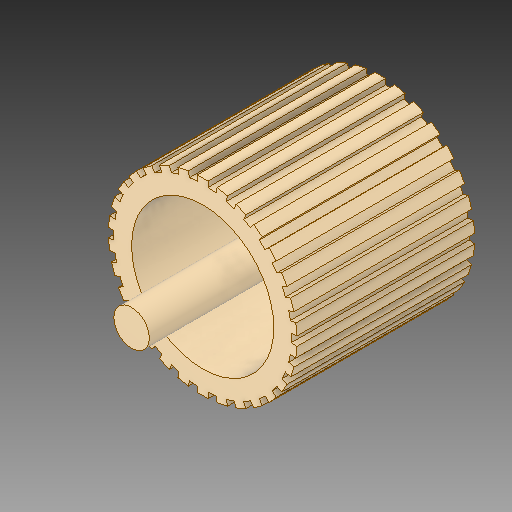
# Autodesk Inventor part: tire
Saved by Autodesk Inventor 2018.1 (Build 221171000, 171)
## iProperties
Created: 2017-10-26
Part Number: tire
Material: 一般
Document SubType Name: Modeling
Designer: Kakeru Yamashita
Density: 28.0819 g/cm^3
Appearance: 滑らか - オフホワイト
Mass: 2000 g
Surface Area: 220.268 cm^2
Volume: 71.2202 cm^3
Author: Kakeru Yamashita
Autodesk Inventor part; units mm, degrees
ref_plane "YZ Plane" through (0, 0, 0) normal (1, 0, 0) x (0, 1, 0)
ref_plane "XZ Plane" through (0, 0, 0) normal (0, 1, 0) x (-1, 0, 0)
ref_plane "XY Plane" through (0, 0, 0) normal (0, 0, 1) x (1, 0, 0)
sketch "スケッチ1" plane through (0, 0, 0) normal (0, 0, 1) x (1, 0, 0)
  line L0 (-37.1163, 0) -> (37.1163, 0) projected
  line L1 (0, -37.1) -> (0, 37.1) projected
  line L2 (1.5, 23.5) -> (1.5, 26.5)
  line L3 (1.5, 26.5) -> (-1.5, 26.5)
  line L4 (-1.5, 26.5) -> (-1.5, 23.5)
  line L5 (-1.5, 23.5) -> (1.5, 23.5)
  line L6 (1.5, 23.5) -> (-1.5, 26.5) construction
  line L7 (1.5, 26.5) -> (-1.5, 23.5) construction
  line L8 (-6.9769, 25.609) -> (-6.3531, 22.6746)
  line L9 (-4.0424, 26.2328) -> (-6.9769, 25.609)
  line L10 (-3.4187, 23.2983) -> (-4.0424, 26.2328)
  line L11 (-6.3531, 22.6746) -> (-3.4187, 23.2983)
  line L12 (-12.1488, 23.5988) -> (-10.9286, 20.8582)
  line L13 (-9.4082, 24.8191) -> (-12.1488, 23.5988)
  line L14 (-8.188, 22.0784) -> (-9.4082, 24.8191)
  line L15 (-10.9286, 20.8582) -> (-8.188, 22.0784)
  line L16 (-16.7898, 20.5573) -> (-15.0265, 18.1302)
  line L17 (-14.3628, 22.3206) -> (-16.7898, 20.5573)
  line L18 (-12.5994, 19.8936) -> (-14.3628, 22.3206)
  line L19 (-15.0265, 18.1302) -> (-12.5994, 19.8936)
  line L20 (-20.697, 16.6172) -> (-18.4676, 14.6099)
  line L21 (-18.6896, 18.8467) -> (-20.697, 16.6172)
  line L22 (-16.4602, 16.8393) -> (-18.6896, 18.8467)
  line L23 (-18.4676, 14.6099) -> (-16.4602, 16.8393)
  line L24 (-23.6997, 11.951) -> (-21.1016, 10.451)
  line L25 (-22.1997, 14.549) -> (-23.6997, 11.951)
  line L26 (-19.6016, 13.049) -> (-22.1997, 14.549)
  line L27 (-21.1016, 10.451) -> (-19.6016, 13.049)
  line L28 (-25.6665, 6.7624) -> (-22.8134, 5.8353)
  line L29 (-24.7395, 9.6155) -> (-25.6665, 6.7624)
  line L30 (-21.8863, 8.6885) -> (-24.7395, 9.6155)
  line L31 (-22.8134, 5.8353) -> (-21.8863, 8.6885)
  line L32 (-26.5116, 1.2782) -> (-23.5281, 0.9646)
  line L33 (-26.198, 4.2618) -> (-26.5116, 1.2782)
  line L34 (-23.2145, 3.9482) -> (-26.198, 4.2618)
  line L35 (-23.5281, 0.9646) -> (-23.2145, 3.9482)
  line L36 (-26.198, -4.2618) -> (-23.2145, -3.9482)
  line L37 (-26.5116, -1.2782) -> (-26.198, -4.2618)
  line L38 (-23.5281, -0.9646) -> (-26.5116, -1.2782)
  line L39 (-23.2145, -3.9482) -> (-23.5281, -0.9646)
  line L40 (-24.7395, -9.6155) -> (-21.8863, -8.6885)
  line L41 (-25.6665, -6.7624) -> (-24.7395, -9.6155)
  line L42 (-22.8134, -5.8353) -> (-25.6665, -6.7624)
  line L43 (-21.8863, -8.6885) -> (-22.8134, -5.8353)
  line L44 (-22.1997, -14.549) -> (-19.6016, -13.049)
  line L45 (-23.6997, -11.951) -> (-22.1997, -14.549)
  line L46 (-21.1016, -10.451) -> (-23.6997, -11.951)
  line L47 (-19.6016, -13.049) -> (-21.1016, -10.451)
  line L48 (-18.6896, -18.8467) -> (-16.4602, -16.8393)
  line L49 (-20.697, -16.6172) -> (-18.6896, -18.8467)
  line L50 (-18.4676, -14.6099) -> (-20.697, -16.6172)
  line L51 (-16.4602, -16.8393) -> (-18.4676, -14.6099)
  line L52 (-14.3628, -22.3206) -> (-12.5994, -19.8936)
  line L53 (-16.7898, -20.5573) -> (-14.3628, -22.3206)
  line L54 (-15.0265, -18.1302) -> (-16.7898, -20.5573)
  line L55 (-12.5994, -19.8936) -> (-15.0265, -18.1302)
  line L56 (-9.4082, -24.8191) -> (-8.188, -22.0784)
  line L57 (-12.1488, -23.5988) -> (-9.4082, -24.8191)
  line L58 (-10.9286, -20.8582) -> (-12.1488, -23.5988)
  line L59 (-8.188, -22.0784) -> (-10.9286, -20.8582)
  line L60 (-4.0424, -26.2328) -> (-3.4187, -23.2983)
  line L61 (-6.9769, -25.609) -> (-4.0424, -26.2328)
  line L62 (-6.3531, -22.6746) -> (-6.9769, -25.609)
  line L63 (-3.4187, -23.2983) -> (-6.3531, -22.6746)
  line L64 (1.5, -26.5) -> (1.5, -23.5)
  line L65 (-1.5, -26.5) -> (1.5, -26.5)
  line L66 (-1.5, -23.5) -> (-1.5, -26.5)
  line L67 (1.5, -23.5) -> (-1.5, -23.5)
  line L68 (6.9769, -25.609) -> (6.3531, -22.6746)
  line L69 (4.0424, -26.2328) -> (6.9769, -25.609)
  line L70 (3.4187, -23.2983) -> (4.0424, -26.2328)
  line L71 (6.3531, -22.6746) -> (3.4187, -23.2983)
  line L72 (12.1488, -23.5988) -> (10.9286, -20.8582)
  line L73 (9.4082, -24.8191) -> (12.1488, -23.5988)
  line L74 (8.188, -22.0784) -> (9.4082, -24.8191)
  line L75 (10.9286, -20.8582) -> (8.188, -22.0784)
  line L76 (16.7898, -20.5573) -> (15.0265, -18.1302)
  line L77 (14.3628, -22.3206) -> (16.7898, -20.5573)
  line L78 (12.5994, -19.8936) -> (14.3628, -22.3206)
  line L79 (15.0265, -18.1302) -> (12.5994, -19.8936)
  line L80 (20.697, -16.6172) -> (18.4676, -14.6099)
  line L81 (18.6896, -18.8467) -> (20.697, -16.6172)
  line L82 (16.4602, -16.8393) -> (18.6896, -18.8467)
  line L83 (18.4676, -14.6099) -> (16.4602, -16.8393)
  line L84 (23.6997, -11.951) -> (21.1016, -10.451)
  line L85 (22.1997, -14.549) -> (23.6997, -11.951)
  line L86 (19.6016, -13.049) -> (22.1997, -14.549)
  line L87 (21.1016, -10.451) -> (19.6016, -13.049)
  line L88 (25.6665, -6.7624) -> (22.8134, -5.8353)
  line L89 (24.7395, -9.6155) -> (25.6665, -6.7624)
  line L90 (21.8863, -8.6885) -> (24.7395, -9.6155)
  line L91 (22.8134, -5.8353) -> (21.8863, -8.6885)
  line L92 (26.5116, -1.2782) -> (23.5281, -0.9646)
  line L93 (26.198, -4.2618) -> (26.5116, -1.2782)
  line L94 (23.2145, -3.9482) -> (26.198, -4.2618)
  line L95 (23.5281, -0.9646) -> (23.2145, -3.9482)
  line L96 (26.198, 4.2618) -> (23.2145, 3.9482)
  line L97 (26.5116, 1.2782) -> (26.198, 4.2618)
  line L98 (23.5281, 0.9646) -> (26.5116, 1.2782)
  line L99 (23.2145, 3.9482) -> (23.5281, 0.9646)
  line L100 (24.7395, 9.6155) -> (21.8863, 8.6885)
  line L101 (25.6665, 6.7624) -> (24.7395, 9.6155)
  line L102 (22.8134, 5.8353) -> (25.6665, 6.7624)
  line L103 (21.8863, 8.6885) -> (22.8134, 5.8353)
  line L104 (22.1997, 14.549) -> (19.6016, 13.049)
  line L105 (23.6997, 11.951) -> (22.1997, 14.549)
  line L106 (21.1016, 10.451) -> (23.6997, 11.951)
  line L107 (19.6016, 13.049) -> (21.1016, 10.451)
  line L108 (18.6896, 18.8467) -> (16.4602, 16.8393)
  line L109 (20.697, 16.6172) -> (18.6896, 18.8467)
  line L110 (18.4676, 14.6099) -> (20.697, 16.6172)
  line L111 (16.4602, 16.8393) -> (18.4676, 14.6099)
  line L112 (14.3628, 22.3206) -> (12.5994, 19.8936)
  line L113 (16.7898, 20.5573) -> (14.3628, 22.3206)
  line L114 (15.0265, 18.1302) -> (16.7898, 20.5573)
  line L115 (12.5994, 19.8936) -> (15.0265, 18.1302)
  line L116 (9.4082, 24.8191) -> (8.188, 22.0784)
  line L117 (12.1488, 23.5988) -> (9.4082, 24.8191)
  line L118 (10.9286, 20.8582) -> (12.1488, 23.5988)
  line L119 (8.188, 22.0784) -> (10.9286, 20.8582)
  line L120 (4.0424, 26.2328) -> (3.4187, 23.2983)
  line L121 (6.9769, 25.609) -> (4.0424, 26.2328)
  line L122 (6.3531, 22.6746) -> (6.9769, 25.609)
  line L123 (3.4187, 23.2983) -> (6.3531, 22.6746)
  arc A0 (-6.6556, 24.0978) -> (-8.7798, 23.4076) centre (0, 0) ccw
  arc A1 (-11.5204, 22.1874) -> (-13.4546, 21.0707) centre (0, 0) ccw
  arc A2 (-15.8817, 19.3073) -> (-17.5415, 17.8128) centre (0, 0) ccw
  arc A3 (-19.5488, 15.5834) -> (-20.8616, 13.7765) centre (0, 0) ccw
  arc A4 (-22.3616, 11.1784) -> (-23.2701, 9.1381) centre (0, 0) ccw
  arc A5 (-24.1971, 6.2849) -> (-24.6615, 4.1003) centre (0, 0) ccw
  arc A6 (-24.975, 1.1167) -> (-24.975, -1.1167) centre (0, 0) ccw
  arc A7 (-24.6615, -4.1003) -> (-24.1971, -6.2849) centre (0, 0) ccw
  arc A8 (-23.2701, -9.1381) -> (-22.3616, -11.1784) centre (0, 0) ccw
  arc A9 (-1.5, 24.955) -> (-3.7212, 24.7215) centre (0, 0) ccw
  arc A10 (3.7212, 24.7215) -> (1.5, 24.955) centre (0, 0) ccw
  arc A11 (8.7798, 23.4076) -> (6.6556, 24.0978) centre (0, 0) ccw
  arc A12 (13.4546, 21.0707) -> (11.5204, 22.1874) centre (0, 0) ccw
  arc A13 (17.5415, 17.8128) -> (15.8817, 19.3073) centre (0, 0) ccw
  arc A14 (20.8616, 13.7765) -> (19.5488, 15.5834) centre (0, 0) ccw
  arc A15 (23.2701, 9.1381) -> (22.3616, 11.1784) centre (0, 0) ccw
  arc A16 (24.6615, 4.1003) -> (24.1971, 6.2849) centre (0, 0) ccw
  arc A17 (24.975, -1.1167) -> (24.975, 1.1167) centre (0, 0) ccw
  arc A18 (24.1971, -6.2849) -> (24.6615, -4.1003) centre (0, 0) ccw
  arc A19 (22.3616, -11.1784) -> (23.2701, -9.1381) centre (0, 0) ccw
  arc A20 (19.5488, -15.5834) -> (20.8616, -13.7765) centre (0, 0) ccw
  arc A21 (15.8817, -19.3073) -> (17.5415, -17.8128) centre (0, 0) ccw
  arc A22 (11.5204, -22.1874) -> (13.4546, -21.0707) centre (0, 0) ccw
  arc A23 (6.6556, -24.0978) -> (8.7798, -23.4076) centre (0, 0) ccw
  arc A24 (1.5, -24.955) -> (3.7212, -24.7215) centre (0, 0) ccw
  arc A25 (-3.7212, -24.7215) -> (-1.5, -24.955) centre (0, 0) ccw
  arc A26 (-8.7798, -23.4076) -> (-6.6556, -24.0978) centre (0, 0) ccw
  arc A27 (-13.4546, -21.0707) -> (-11.5204, -22.1874) centre (0, 0) ccw
  arc A28 (-20.8616, -13.7765) -> (-19.5488, -15.5834) centre (0, 0) ccw
  arc A29 (-17.5415, -17.8128) -> (-15.8817, -19.3073) centre (0, 0) ccw
  point P0 (0, 25)
  dimension "d1" = 3
  dimension "d2" = 3
  dimension "d5" = 360
  constraints: 244 end point, 61 point on line, 3 parallel, 2 midpoint, 2 vertical alignment, 1 perpendicular, 330 other
  measures "d1" distance of L2.end L3.end
  measures "d2" distance between parallel lines of L5 L3
extrude "押し出し1" add sketch "スケッチ1" along normal blind 50
sketch "スケッチ2" plane through (0, 0, 50) normal (0, 0, 1) x (1, 0, 0)
  circle A0 centre (0, 0) radius 20
  dimension "d9" = 40
  constraints: 1 centre point, 1 coincident
  measures "d9" diameter of A0
extrude "押し出し2" cut sketch "スケッチ2" against normal blind 30
sketch "スケッチ3" plane through (0, 0, 20) normal (0, 0, 1) x (1, 0, 0)
  circle A0 centre (0, 0) radius 5
  dimension "d12" = 10
  constraints: 1 centre point, 1 coincident
  measures "d12" diameter of A0
extrude "押し出し3" add sketch "スケッチ3" along normal blind 50
